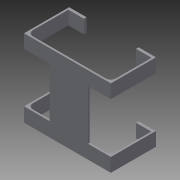
# Autodesk Inventor part: tapa
Saved by Autodesk Inventor 2013 (Build 170138000, 138)
## iProperties
Created: 2013-05-01
Part Number: tapa
Material: Generic
Document SubType Name: Modeling
Designer: otrab
Density: 1 g/cm^3
Author: otrab
Autodesk Inventor part; units mm, degrees
ref_plane "YZ Plane" through (0, 0, 0) normal (1, 0, 0) x (0, 1, 0)
ref_plane "XZ Plane" through (0, 0, 0) normal (0, 1, 0) x (-1, 0, 0)
ref_plane "XY Plane" through (0, 0, 0) normal (0, 0, 1) x (1, 0, 0)
sketch "Sketch1" plane through (0, 0, 0) normal (0, 1, 0) x (-1, 0, 0)
  line L0 (-25, -31) -> (25, -31)
  line L1 (25, -31) -> (25, 31)
  line L2 (25, 31) -> (-25, 31)
  line L3 (-25, 31) -> (-25, -31)
  line L4 (-25, -31) -> (25, 31) construction
  line L5 (25, -31) -> (-25, 31) construction
  point P0 (0, 0)
  dimension "d0" = 50
  dimension "d2" = 62
  constraints: 12 end point, 2 midpoint, 2 parallel, 1 horizontal, 1 perpendicular
  measures "d0" distance of L1.end L2.end
  measures "d2" distance of L2.end L0.start
extrude "Extrusion1" add sketch "Sketch1" along normal blind 1
sketch "Sketch2" plane through (0, 1, 0) normal (0, 1, 0) x (1, 0, 0)
  line L0 (25, 31) -> (-25, 31) projected
  line L1 (-25, 31) -> (-25, -31) projected
  line L2 (-25, -31) -> (25, -31) projected
  line L3 (-25, 31) -> (-24, 31)
  line L4 (-24, 31) -> (-24, -31)
  line L5 (-25, -31) -> (-24, -31)
  line L6 (-25, -31) -> (-25, 31)
  line L7 (0, 46.5401) -> (0, -49.8176) construction
  line L8 (25, 31) -> (25, -31)
  line L9 (25, 31) -> (24, 31)
  line L10 (24, 31) -> (24, -31)
  line L11 (25, -31) -> (24, -31)
  line L12 (25, -31) -> (25, 31)
  point P0 (0, 0)
  dimension "d5" = 1
  constraints: 20 end point, 3 perpendicular, 2 point on line, 2 symmetric about line, 1 parallel
  measures "d5" distance of L0.end L3.end
extrude "Extrusion2" add sketch "Sketch2" along normal blind 22 contours L8 L2 L10 L0 | L4 L2 L1 L0
fillet "Fillet1" radius 3 1 edges at (-24, 1, 0)
mirror "Mirror1" about plane through (0, 0, 0) normal (1, 0, 0) of "Fillet1"
sketch "Sketch3" plane through (-25, 0, -31) normal (-1, 0, 0) x (0, 0, 1)
  line L0 (0, 0) -> (62, 0) projected
  line L1 (62, 23) -> (61, 23) construction
  line L2 (61, 23) -> (61, 21.5)
  line L3 (61, 21.5) -> (53, 21.5)
  line L4 (53, 21.5) -> (53, 23)
  line L5 (61, 23) -> (53, 23)
  line L6 (53, 23) -> (61, 23)
  point P0 (31, 0)
  dimension "d9" = 1
  dimension "d10" = 1.5
  dimension "d11" = 8
  constraints: 12 end point, 1 parallel, 1 perpendicular
  measures "d9" distance of L1.start L1.end
  measures "d10" distance of L1.end L2.end
  measures "d11" distance of L2.end L3.end
extrude "Extrusion3" add sketch "Sketch3" against normal blind 7
mirror "Mirror3" about plane through (0, 0, 0) normal (0, 0, 1) of "Extrusion3"
mirror "Mirror4" about plane through (0, 0, 0) normal (1, 0, 0) of "Extrusion3", "Mirror3"
sketch "Sketch6" plane through (0, 23, 0) normal (0, 1, 0) x (1, 0, 0)
  line L0 (-30.2809, -30.0039) -> (31.8564, -30.0039)
  line L1 (31.8564, -30.0039) -> (31.8564, -41.1164)
  line L2 (31.8564, -41.1164) -> (-30.2809, -41.1164)
  line L3 (-30.2809, -41.1164) -> (-30.2809, -30.0039)
  line L4 (-30.2809, 39.7218) -> (31.1002, 39.7218)
  line L5 (31.1002, 39.7218) -> (31.1002, 30.1983)
  line L6 (31.1002, 30.1983) -> (-30.2809, 30.1983)
  line L7 (-30.2809, 30.1983) -> (-30.2809, 39.7218)
  line L8 (-30.2809, 22.0008) -> (-10.2809, 22.0008)
  line L9 (-10.2809, 22.0008) -> (-10.2809, -21.9612)
  line L10 (-10.2809, -21.9612) -> (-30.2809, -21.9612)
  line L11 (-30.2809, -21.9612) -> (-30.2809, 22.0008)
  line L12 (31.8564, -21.9503) -> (11.8564, -21.9503)
  line L13 (11.8564, -21.9503) -> (11.8564, 22.0008)
  line L14 (11.8564, 22.0008) -> (31.8564, 22.0008)
  line L15 (31.8564, 22.0008) -> (31.8564, -21.9503)
  point P0 (0, 0)
  dimension "d26" = 20
  dimension "d27" = 20
  constraints: 32 end point, 8 parallel, 4 horizontal, 4 perpendicular, 1 collinear
  measures "d26" distance of L9.end L10.end
  measures "d27" distance of L13.end L14.end
extrude "Extrusion6" cut sketch "Sketch6" against normal through all
body "Solid1"
